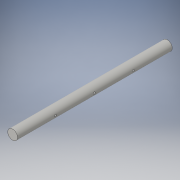
# Autodesk Inventor part: Straw
Saved by Autodesk Inventor 2016 (Build 200138000, 138)
## iProperties
Created: 2017-04-26
Part Number: Straw
Material: Generic
Document SubType Name: Modeling
Designer: wtse3759
Density: 1 g/cm^3
Appearance: Default
Author: wtse3759
Autodesk Inventor part; units mm, degrees
ref_plane "YZ Plane" through (0, 0, 0) normal (1, 0, 0) x (0, 1, 0)
ref_plane "XZ Plane" through (0, 0, 0) normal (0, 1, 0) x (-1, 0, 0)
ref_plane "XY Plane" through (0, 0, 0) normal (0, 0, 1) x (1, 0, 0)
sketch "Sketch1" plane through (0, 0, 0) normal (0, 0, 1) x (1, 0, 0)
  circle A0 centre (0, 0) radius 6.35
  dimension "d0" = 12.7
  constraints: 1 centre point, 1 coincident
  measures "d0" diameter of A0
extrude "Extrusion1" add sketch "Sketch1" along normal blind 203.2
sketch "Sketch5" plane through (0, 0, 0) normal (0, 1, 0) x (-1, 0, 0)
  line L0 (0, 1.524) -> (-1.27, 1.524)
  line L1 (-6.35, 0) -> (6.35, 0) projected
  line L2 (-1.27, 0) -> (1.27, 0)
  line L3 (1.27, 1.524) -> (0, 1.524)
  line L4 (1.27, 1.524) -> (6.35, 1.524)
  line L5 (6.35, 0) -> (6.35, 203.2) projected
  line L6 (6.35, 1.524) -> (-6.35, 1.524)
  line L7 (-6.35, 1.524) -> (-6.35, 0)
  line L8 (-6.35, 0) -> (6.35, 0)
  line L9 (6.35, 0) -> (6.35, 1.524)
  line L10 (6.35, 203.2) -> (-6.35, 203.2) projected
  line L11 (-6.35, 203.2) -> (6.35, 203.2)
  line L12 (6.35, 203.2) -> (6.35, 201.676)
  line L13 (6.35, 201.676) -> (-6.35, 201.676)
  line L14 (-6.35, 201.676) -> (-6.35, 203.2)
  point P0 (0, 0)
  dimension "d20" = 1.524
  dimension "d21" = 1.27
  dimension "d26" = 12.7
  dimension "d27" = 1.524
  constraints: 24 end point, 5 equal length, 4 point on line, 3 horizontal, 2 perpendicular
  measures "d20" distance of point (0, 0) L0.start
  measures "d21" distance of L0.start L0.end
  measures "d26" distance of L12.end L13.end
  measures "d27" distance of L11.end L12.end
sketch "Sketch7" plane through (0, 0, 0) normal (1, 0, 0) x (0, 1, 0)
  line L0 (0, 0) -> (0, 50.8)
  circle A0 centre (0, 50.8) radius 1.27
  line L1 (0, 50.8) -> (0, 101.6)
  circle A1 centre (0, 101.6) radius 1.27
  line L2 (0, 101.6) -> (0, 152.4)
  circle A2 centre (0, 152.4) radius 1.27
  dimension "d42" = 50.8
  dimension "d43" = 2.54
  dimension "d44" = 50.8
  dimension "d45" = 2.54
  dimension "d46" = 50.8
  dimension "d47" = 2.54
  constraints: 6 end point, 3 centre point, 3 coincident, 3 vertical
  measures "d42" distance of L0.start L0.end
  measures "d43" diameter of A0
  measures "d44" distance of L1.start L1.end
  measures "d45" diameter of A1
  measures "d46" distance of L2.start L2.end
  measures "d47" diameter of A2
extrude "Extrusion8" cut sketch "Sketch7" along normal mid plane 25.4
extrude "Extrusion9" cut sketch "Sketch5" along normal mid plane 25.4 contours L13 L14 L10 L5
body "Solid1"
